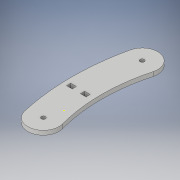
# Autodesk Inventor part: fem2
Saved by Autodesk Inventor 2019 (Build 230136000, 136)
## iProperties
Created: 2023-04-15
Part Number: fem2
Material: Generic
Document SubType Name: Modeling
Designer: Analuam
Density: 1 g/cm^3
Appearance: Default
Author: Analuam
Autodesk Inventor part; units mm, degrees
ref_plane "YZ Plane" through (0, 0, 0) normal (1, 0, 0) x (0, 1, 0)
ref_plane "XZ Plane" through (0, 0, 0) normal (0, 1, 0) x (-1, 0, 0)
ref_plane "XY Plane" through (0, 0, 0) normal (0, 0, 1) x (1, 0, 0)
sketch "Sketch1" plane through (0, 0, 0) normal (0, 1, 0) x (-1, 0, 0)
  arc A0 (13.7652, 13.7563) -> (-7.6488, 8.7996) centre (2.9529, 11.7331) ccw
  arc A1 (-7.6488, -55.3335) -> (13.7652, -60.2902) centre (2.9529, -58.2669) ccw
  arc A2 (-7.6723, -55.4199) -> (-7.6723, 8.8861) centre (-125.5725, -23.2669) ccw
  arc A3 (13.578, -61.1139) -> (13.578, 14.5801) centre (-151.1069, -23.2669) ccw
  circle A4 centre (2.9529, 11.7331) radius 1.5
  circle A5 centre (2.9529, -58.2669) radius 1.5
  line L0 (14.3609, -16.1047) -> (10.3609, -16.1047)
  line L1 (10.3609, -16.1047) -> (10.3609, -19.1047)
  line L2 (10.3609, -19.1047) -> (14.3609, -19.1047)
  line L3 (14.3609, -19.1047) -> (14.3609, -16.1047)
  line L4 (14.3609, -11.7669) -> (10.3609, -14.7669) construction
  line L5 (10.3609, -11.7669) -> (14.3609, -14.7669) construction
  line L6 (0.5448, -16.1047) -> (4.5448, -16.1047)
  line L7 (4.5448, -16.1047) -> (4.5448, -19.1047)
  line L8 (4.5448, -19.1047) -> (0.5448, -19.1047)
  line L9 (0.5448, -19.1047) -> (0.5448, -16.1047)
  line L10 (12.3609, -13.2669) -> (12.3609, -13.2669)
  line L11 (2.9529, 11.7331) -> (2.9529, -58.2669)
  line L12 (10.3609, -18.6047) -> (4.5448, -18.6047)
  line L13 (7.4529, -18.6047) -> (7.4529, -17.6047)
  point P0 (0, 0)
  dimension "d0" = 22
  dimension "d1" = 22
  dimension "d2" = 70
  dimension "d3" = 3
  dimension "d4" = 3
  dimension "d21" = 4
  dimension "d22" = 3
  dimension "d25" = 0
  dimension "d26" = 1
  constraints: 28 end point, 16 point on circle, 6 centre point, 3 vertical, 2 coincident, 2 parallel, 1 horizontal, 1 midpoint, 1 perpendicular
  measures "d0" diameter of A0
  measures "d1" diameter of A1
  measures "d2" distance of A1.centre A0.centre
  measures "d3" diameter of A4
  measures "d4" diameter of A5
  measures "d21" distance of L2.end L1.end
  measures "d22" distance of L1.end L0.end
  measures "d25" distance of L10.start L10.end
  measures "d26" distance of L13.start L13.end
sketch "Sketch2" plane through (0, 0, 0) normal (0, 1, 0) x (-1, 0, 0)
  point P0 (0, 0)
extrude "Extrusion1" add sketch "Sketch1" along normal blind 3 contours A3 A1 A2 A0
sketch "Sketch3" plane through (0, 0, 0) normal (0, -1, 0) x (1, 0, 0)
  point P0 (0, 0)
sketch "Sketch4" plane through (0, 0, 0) normal (0, -1, 0) x (1, 0, 0)
  point P0 (0, 0)
sketch "Sketch5" plane through (0, 3, 0) normal (0, 1, 0) x (1, 0, 0)
  point P0 (0, 0)
sketch "Sketch6" plane through (0, 3, 0) normal (0, 1, 0) x (1, 0, 0)
  point P0 (0, 0)
body "Solid1"
